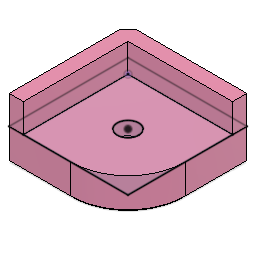
Bed Build Plate Alignment Stops v5 (Autodesk Fusion 360 archive; units mm, degrees)
design "Bed Build Plate Alignment Stops" references "Bed Build Plate Alignment Stops"
Autodesk Fusion 360 part; units mm, degrees
sketch "Sketch1" plane through (0, 0, 0) normal (0, 1, 0) x (1, 0, 0)
  circle A0 centre (10, -10) radius 2.25
  line L0 (-3, 3) -> (22, 3)
  line L1 (-3, 3) -> (-3, -22)
  line L2 (0, 0) -> (22, 0)
  line L3 (22, 0) -> (22, -22)
  line L4 (22, -22) -> (0, -22)
  line L5 (0, -22) -> (0, 0)
  line L6 (22, 3) -> (22, 0)
  line L7 (-3, -22) -> (0, -22)
  dimension "d1" = 4.5
  dimension "d2" = 10
  dimension "d3" = 10
  dimension "d4" = 3
  dimension "d5" = 3
  dimension "d6" = 22
  dimension "d7" = 22
  dimension "d8" = 25
  dimension "d9" = 25
  constraint horizontal L0
  constraint perpendicular L0 L1
  constraint horizontal L2
  constraint vertical L3
  constraint horizontal L4
  constraint vertical L5
  constraint coincident L2.start L5.end
  measures "d1" diameter of A0
  measures "d2" distance of L2.start A0.centre
  measures "d3" distance of L2.start A0.centre
  measures "d4" distance of L2.start L1
  measures "d5" distance of L2.start L0
  measures "d6" distance of L2.start L2.end
  measures "d7" distance of L2.start L4.end
  measures "d8" distance of L0.start L0.end
  measures "d9" distance of L0.start L1.end
extrude "Extrude1" add sketch "Sketch1" along normal blind 6 contours L0 L1 L2 L5 L6 L7
extrude "Extrude2" add sketch "Sketch1" against normal blind 3.2
chamfer "Chamfer1" distance 1.6 angle 45 1 edges at (-3, 1.4, -3)
fillet "Fillet1" radius 12 1 edges at (22, -1.6, 22)
sketch "Sketch2" plane through (0, -3.2, 0) normal (0, -1, 0) x (1, 0, 0)
  circle A0 centre (10, 10) radius 2.25
  arc A1 (22, 10) -> (10, 22) centre (10, 10) ccw
  line L0 (10, 22) -> (-3, 22)
  line L1 (-3, 22) -> (-3, -1.4)
  line L2 (-3, -1.4) -> (-1.4, -3)
  line L3 (-1.4, -3) -> (22, -3)
  line L4 (22, -3) -> (22, 10)
  circle A2 centre (10, 10) radius 2.25
  line L5 (10, 5.9585) -> (13.5, 7.9793)
  line L6 (13.5, 7.9793) -> (13.5, 12.0207)
  line L7 (13.5, 12.0207) -> (10, 14.0415)
  line L8 (10, 14.0415) -> (6.5, 12.0207)
  line L9 (6.5, 12.0207) -> (6.5, 7.9793)
  line L10 (6.5, 7.9793) -> (10, 5.9585)
  point P0 (10, 10)
  dimension "d17" = 3.5
  constraint coincident P0 A0.centre
  constraint vertical L9
  measures "d17" distance of P0 L10
extrude "Extrude3" add sketch "Sketch2" along normal blind 3.4 contours A1 L0 L1 L2 L3 L4
sketch "Sketch3" plane through (0, -3.2, 0) normal (0, -1, 0) x (1, 0, 0)
  line L0 (10, 5.9585) -> (13.5, 7.9793)
  line L1 (13.5, 7.9793) -> (13.5, 12.0207)
  line L2 (13.5, 12.0207) -> (10, 14.0415)
  line L3 (10, 14.0415) -> (6.5, 12.0207)
  line L4 (6.5, 12.0207) -> (6.5, 7.9793)
  line L5 (6.5, 7.9793) -> (10, 5.9585)
  circle A0 centre (10, 10) radius 2.25
  line L6 (9.6029, 6.1878) -> (6.5, 11.5622)
  line L7 (13.5, 8.4378) -> (10.3971, 13.8122)
  line L8 (13.1029, 7.75) -> (6.8971, 7.75)
  line L9 (13.1029, 12.25) -> (6.8971, 12.25)
  circle A1 centre (10, 10) radius 2.25
  constraint coincident L5 L6.start
  constraint coincident L4 L6.end
  constraint coincident L1 L7.start
  constraint coincident L2 L7.end
  constraint tangent A0 L7
  constraint tangent A0 L6
  constraint perpendicular L0 L7
  constraint perpendicular L0 L6
  constraint coincident L0 L8.start
  constraint coincident L5 L8.end
  constraint coincident L2 L9.start
  constraint coincident L3 L9.end
  constraint perpendicular L4 L8
  constraint perpendicular L4 L9
  constraint tangent L9 A1
  constraint tangent L8 A1
extrude "Extrude4" cut sketch "Sketch3" against normal blind 0.4 contours L0 L1 A0 L7 L8 A1 | A0 L6 L8 A1 | L3 L4 A0 L6 L9 A1 | A0 L7 L9 A1
extrude "Extrude5" cut sketch "Sketch3" against normal blind 0.2 contours L0 L5 L6 L8 | L2 L3 L7 L9
chamfer "Chamfer2" distance 0.4 angle 45 1 faces at (0.1667, -6.6, 10.8736)
equation "d17 = ( 7 / 2 ) * 1 mm"
